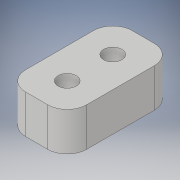
# Autodesk Inventor part: travel_mount
Saved by Autodesk Inventor 2018 (Build 220112000, 112)
## iProperties
Created: 2020-03-14
Part Number: travel_mount
Material: Generic
Document SubType Name: Modeling
Designer: natha
Density: 1 g/cm^3
Appearance: Default
Author: natha
Autodesk Inventor part; units mm, degrees
ref_plane "YZ Plane" through (0, 0, 0) normal (1, 0, 0) x (0, 1, 0)
ref_plane "XZ Plane" through (0, 0, 0) normal (0, 1, 0) x (-1, 0, 0)
ref_plane "XY Plane" through (0, 0, 0) normal (0, 0, 1) x (1, 0, 0)
sketch "Sketch1" plane through (0, 0, 0) normal (0, 1, 0) x (-1, 0, 0)
  line L0 (0, 0) -> (40, 0)
  line L1 (40, 0) -> (40, -70)
  line L2 (40, -70) -> (0, -70)
  line L3 (0, -70) -> (0, 0)
  circle A0 centre (20, -50) radius 6
  circle A1 centre (20, -20) radius 6
  dimension "d0" = 40
  dimension "d1" = 70
  dimension "d2" = 12
  dimension "d3" = 12
  dimension "d4" = 20
  dimension "d5" = 30
  constraints: 8 end point, 2 centre point, 2 parallel, 1 horizontal, 1 perpendicular
  measures "d0" distance of L1.end L2.end
  measures "d1" distance of L0.end L1.end
  measures "d2" diameter of A0
  measures "d3" diameter of A1
  measures "d4" distance from line of L2 A0.centre
  measures "d5" distance of A0.centre A1.centre
extrude "Extrusion1" add sketch "Sketch1" along normal blind 25.4
fillet "Fillet1" radius 12.7 4 edges at (0, 12.7, -70) (-40, 12.7, -70) (0, 12.7, 0) (-40, 12.7, 0)
body "Solid1"
